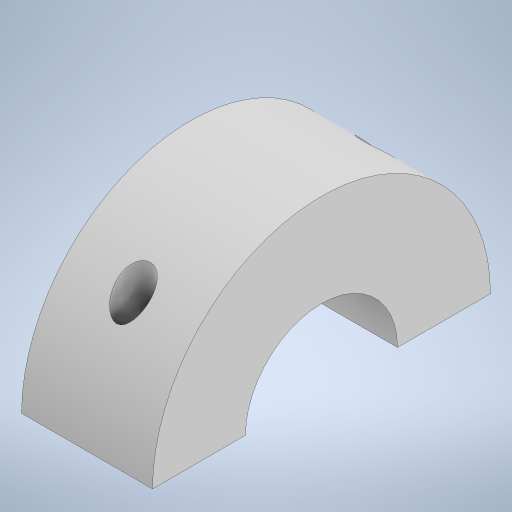
# Autodesk Inventor part: Parte2
Saved by Autodesk Inventor 2023 (Build 270158000, 158)
## iProperties
Created: 2022-11-03
Part Number: Parte2
Material: Generic
Document SubType Name: Modeling
Designer: ivanm
Density: 1 g/cm^3
Appearance: Default
Author: ivanm
Autodesk Inventor part; units mm, degrees
ref_plane "YZ Plane" through (0, 0, 0) normal (1, 0, 0) x (0, 1, 0)
ref_plane "XZ Plane" through (0, 0, 0) normal (0, 1, 0) x (-1, 0, 0)
sketch "Sketch1" plane through (0, 0, 0) normal (1, 0, 0) x (0, 1, 0)
  arc A0 (0, -20) -> (0, 20) centre (0, 0) ccw
  arc A1 (0, -9) -> (0, 9) centre (0, 0) ccw
  line L0 (0, 20) -> (0, 9)
  line L1 (0, -9) -> (0, -20)
  dimension "d0" = 18
  dimension "d1" = 40
  dimension "d10" = 11
  dimension "d11" = 11
  constraints: 4 end point, 4 point on circle, 3 coincident, 2 centre point, 2 vertical
  measures "d0" diameter of A1
  measures "d1" diameter of A0
  measures "d10" distance of L0.start L0.end
  measures "d11" distance of L1.start L1.end
extrude "Extrusion1" add sketch "Sketch1" along normal blind 15.5
ref_plane "Work Plane1" through (0, -20, 0) normal (0, -1, 0) x (1, 0, 0)
sketch "Sketch2" plane through (0, -20, 0) normal (0, -1, 0) x (1, 0, 0)
  line L0 (0, 20) -> (0, 9) projected
  line L1 (0, 9) -> (15.5, 9) projected
  line L2 (15.5, 20) -> (15.5, 9) projected
  line L3 (0, 20) -> (15.5, 20) projected
  line L4 (0, -9) -> (0, -20) projected
  line L5 (0, -20) -> (15.5, -20) projected
  line L6 (15.5, -9) -> (15.5, -20) projected
  line L7 (0, -9) -> (15.5, -9) projected
  circle A0 centre (7.75, 14.5) radius 2
  circle A1 centre (7.75, -14.5) radius 2
  line L8 (15.5, 14.5) -> (0, 14.5) construction
  line L9 (7.75, 9) -> (7.75, 20) construction
  line L10 (7.75, -9) -> (7.75, -20) construction
  line L11 (0, -14.5) -> (15.5, -14.5) construction
  point P0 (0, 0)
  dimension "d6" = 4
  dimension "d7" = 4
  constraints: 10 midpoint, 8 end point, 2 centre point, 2 coincident
  measures "d6" diameter of A0
  measures "d7" diameter of A1
extrude "Extrusion2" cut sketch "Sketch2" against normal through all contours A0 | A1
equation "\"d7\" = d6"
body "Solid1"
